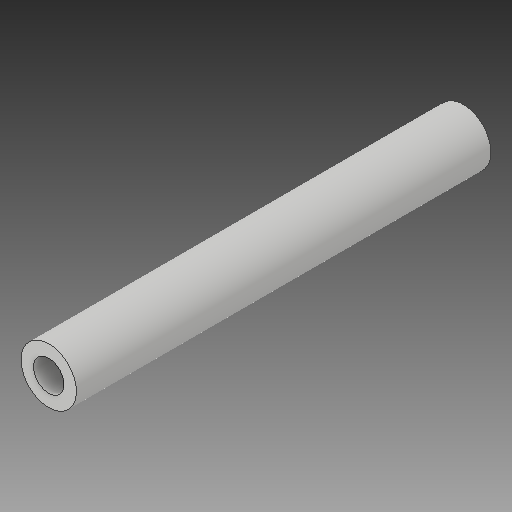
# Autodesk Inventor part: Стойка между первым и вторым этажом
Saved by Autodesk Inventor 2019.1 (Build 231200000, 200)
## iProperties
Created: 2018-06-14
Part Number: Стойка между первым и вторым этажом
Material: Типовые
Document SubType Name: Modeling
Designer: olege
Density: 1 g/cm^3
Appearance: По умолчанию
Mass: 2.10361 g
Surface Area: 24.0747 cm^2
Volume: 2.10361 cm^3
Author: olege
Autodesk Inventor part; units mm, degrees
ref_plane "YZ Plane" through (0, 0, 0) normal (1, 0, 0) x (0, 1, 0)
ref_plane "XZ Plane" through (0, 0, 0) normal (0, 1, 0) x (-1, 0, 0)
ref_plane "XY Plane" through (0, 0, 0) normal (0, 0, 1) x (1, 0, 0)
sketch "Эскиз1" plane through (0, 0, 0) normal (0, 0, 1) x (1, 0, 0)
  circle A0 centre (0, 0) radius 2.2
  circle A1 centre (0, 0) radius 4
  dimension "d0" = 4.4
  dimension "d1" = 8
  constraints: 2 centre point, 2 coincident
  measures "d0" diameter of A0
  measures "d1" diameter of A1
extrude "Выдавливание1" add sketch "Эскиз1" along normal blind 60
